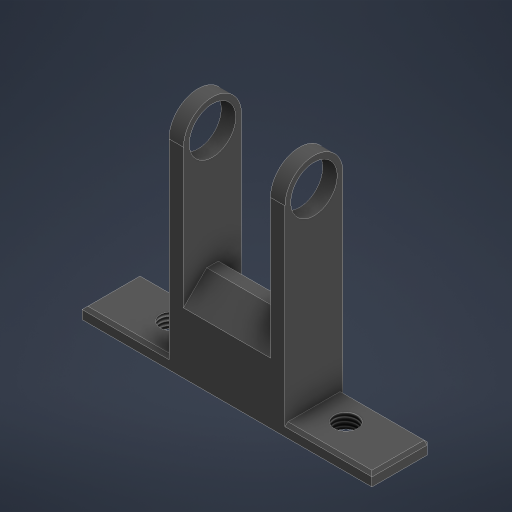
# Autodesk Inventor part: Bearing Block
Saved by Autodesk Inventor 2023 (Build 270158000, 158)
## iProperties
Created: 2021-12-04
Part Number: Bearing Block
Material: Generic
Document SubType Name: Modeling
Designer: LEGION SMIT
Density: 1 g/cm^3
Appearance: Generic
Author: LEGION SMIT
Autodesk Inventor part; units mm, degrees
ref_plane "YZ Plane" through (0, 0, 0) normal (1, 0, 0) x (0, 1, 0)
ref_plane "XZ Plane" through (0, 0, 0) normal (0, 1, 0) x (-1, 0, 0)
ref_plane "XY Plane" through (0, 0, 0) normal (0, 0, 1) x (1, 0, 0)
sketch "Sketch4" plane through (0, 0, 0) normal (0, 0, 1) x (1, 0, 0)
  line L0 (0, 0) -> (-25, 0)
  line L1 (-25, 0) -> (-25, 2.5)
  line L2 (-25, 2.5) -> (-10, 2.5)
  line L3 (-10, 2.5) -> (-10, 40)
  line L4 (-10, 40) -> (-7.5, 40)
  line L5 (-7.5, 40) -> (-7.5, 15)
  line L6 (-7.5, 15) -> (0, 15)
  line L7 (0, 15) -> (0, 0)
  line L8 (0, 0) -> (25, 0)
  line L9 (25, 0) -> (25, 2.5)
  line L10 (25, 2.5) -> (10, 2.5)
  line L11 (10, 2.5) -> (10, 40)
  line L12 (10, 40) -> (7.5, 40)
  line L13 (7.5, 40) -> (7.5, 15)
  line L14 (7.5, 15) -> (0, 15)
  dimension "d43" = 25
  dimension "d44" = 2.5
  dimension "d45" = 15
  dimension "d46" = 37.5
  dimension "d47" = 2.5
  dimension "d48" = 25
  constraints: 30 end point, 6 perpendicular, 6 symmetric about line, 1 horizontal, 1 parallel
  measures "d43" distance of L0.start L0.end
  measures "d44" distance of L0.end L1.end
  measures "d45" distance of L1.end L2.end
  measures "d46" distance of L2.end L3.end
  measures "d47" distance of L3.end L4.end
  measures "d48" distance of L4.end L5.end
extrude "Extrusion3" add sketch "Sketch4" along normal blind 10
fillet "Fillet6" radius 5 4 edges at (8.75, 40, 10) (8.75, 40, 0) (-8.75, 40, 0) (-8.75, 40, 10)
chamfer "Chamfer1" distance 0.5 angle 45 11 edges at (17.5, 2.5, 0) (25, 2.5, 5) (17.5, 2.5, 10) (-17.5, 2.5, 0) (-25, 2.5, 5) (-17.5, 2.5, 10) (-12.5, 0, 0) (-25, 0, 5) (-12.5, 0, 10) (25, 0, 5) (25, 1.25, 0)
sketch "Sketch5" plane through (-24.5, 2.5, 0.5) normal (0, 1, 0) x (1, 0, 0)
  line L0 (0, -9) -> (0, 0) projected
  line L1 (0, 0) -> (14.5, 0) projected
  point P0 (24.5, 0.5)
  point P1 (9.5, -4)
  dimension "d57" = 9.5
  dimension "d58" = 4
  measures "d57" distance from line of L0 point (9.5, -4)
  measures "d58" distance from line of L1 point (9.5, -4)
hole "Hole2" at (-15, 2.5, 4.5) direction (0, -1, 0) diameter 4 end through all
thread "Thread3" size "M4x0.7" class "6H" standard "ANSI Metric M Profile" full length
mirror "Mirror1" about plane through (0, 0, 0) normal (1, 0, 0) of "Hole2"
sketch "Sketch6" plane through (10, 35, 5) normal (1, 0, 0) x (0, 0, -1)
  arc A0 (5, 0) -> (-5, 0) centre (0, 0) ccw projected
  point P0 (5, -35)
  constraints: 1 coincident
hole "Hole3" at (10, 35, 5) direction (-1, 0, 0) diameter 8 end through all
chamfer "Chamfer2" distance 4 angle 45 1 edges at (0, 15, 10)
chamfer "Chamfer3" distance 4 angle 45 1 edges at (0, 15, 0)
body "Solid2"
